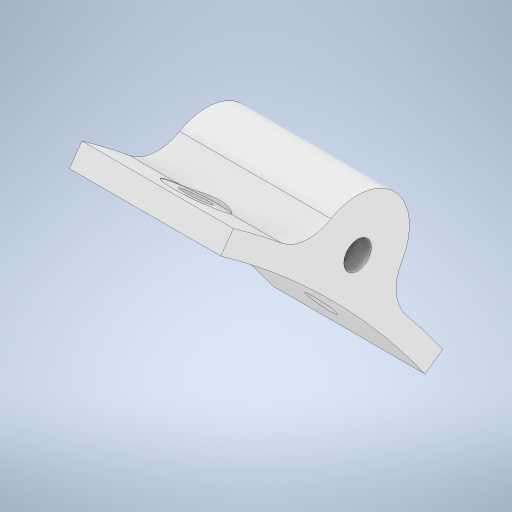
# Autodesk Inventor part: Lüfterhalter
Saved by Autodesk Inventor 2023 (Build 270158000, 158)
## iProperties
Created: 2023-01-25
Part Number: Lüfterhalter
Material: Generisch
Document SubType Name: Modeling
Designer: prigge
Density: 1 g/cm^3
Appearance: Glatt - Weiß
Author: prigge
Autodesk Inventor part; units mm, degrees
ref_plane "XY Plane" through (0, 0, 0) normal (0, 0, 1) x (1, 0, 0)
sketch "Skizze1" plane through (0, 0, 0) normal (1, 0, 0) x (0, 1, 0)
  line L0 (0, 0) -> (147.4318, -147.4318) construction
  line L1 (0, 33.4705) -> (0, -200.8229) construction
  circle A0 centre (147.4318, -147.4318) radius 3.2
  line L2 (0, 0) -> (156.5216, -124.5029) construction
  line L3 (-33.4705, 0) -> (200.8229, 0) projected
  arc A1 (115.8562, -163.0256) -> (163.0256, -115.8562) centre (0, 0) ccw
  line L4 (0, 0) -> (163.0256, -115.8562) construction
  line L5 (163.0256, -115.8562) -> (167.1012, -118.7526)
  arc A2 (152.7783, -136.6887) -> (167.1012, -118.7526) centre (0, 0) ccw
  arc A3 (118.7526, -167.1012) -> (136.6887, -152.7783) centre (0, 0) ccw
  arc A4 (136.6887, -152.7783) -> (152.7783, -136.6887) centre (147.4318, -147.4318) ccw
  line L6 (115.8562, -163.0256) -> (118.7526, -167.1012)
  dimension "d0" = 45
  dimension "d1" = 208.5
  dimension "d2" = 6.4
  dimension "d3" = 38.5
  dimension "d4" = 200
  dimension "d5" = 54.6
  dimension "d6" = 5
  dimension "d7" = 12
  constraints: 10 end point, 10 point on circle, 5 centre point, 3 coincident, 3 symmetric about line, 2 point on line, 1 collinear, 1 other
  measures "d0" angle of L1 L0
  measures "d1" distance of L0.start L0.end
  measures "d2" diameter of A0
  measures "d3" angle of L3 L2
  measures "d4" radius of A1
  measures "d5" angle of L1 L4
  measures "d6" distance of L4.end L5.end
  measures "d7" radius of A4
extrude "Extrusion1" add sketch "Skizze1" against normal blind 35
fillet "Rundung1" radius 10 2 edges at (-17.5, 136.6887, -152.7783) (-17.5, 152.7783, -136.6887)
ref_plane "Arbeitsebene1" through (-17.5, 0, 0) normal (1, 0, 0) x (0, 1, 0)
sketch "Skizze2" plane through (-17.5, 0, 0) normal (1, 0, 0) x (0, 1, 0)
  line L0 (0, 0) -> (141.692, -178.1312) construction
  line L1 (0, -213.7575) -> (0, 35.6262) projected
  line L2 (124.487, -156.5016) -> (121.9826, -158.4936)
  arc A0 (115.8562, -163.0256) -> (163.0256, -115.8562) centre (0, 0) ccw projected
  line L3 (121.9826, -158.4936) -> (125.047, -162.3461)
  arc A1 (118.7526, -167.1012) -> (129.8706, -158.6147) centre (0, 0) ccw projected
  line L4 (125.047, -162.3461) -> (122.4644, -164.4004)
  line L5 (122.4644, -164.4004) -> (125.577, -168.3134)
  line L6 (125.577, -168.3134) -> (130.6639, -164.267)
  line L7 (124.487, -156.5016) -> (130.6639, -164.267)
  point P0 (124.5029, -156.5216)
  dimension "d12" = 38.5
  dimension "d13" = 5
  dimension "d14" = 6.4
  dimension "d15" = 13
  constraints: 14 end point, 4 perpendicular, 2 point on circle, 2 point on line, 1 collinear, 1 parallel
  measures "d12" angle of L1 L0
  measures "d13" distance of L4.end L5.end
  measures "d14" diameter of L3 L0
  measures "d15" diameter of L5 L0
revolve "Umdrehung1" cut sketch "Skizze2" angle 360 about axis through (-17.5, 0, 0) along (0, 0.6225146, -0.7826082) contours A0 L7 A1 L4 L3 | L7 L6 L5 A1
ref_plane "Arbeitsebene2" through (0, 0, 0) normal (0, 0.7071068, 0.7071068) x (1, 0, 0)
mirror "Spiegeln1" about plane through (0, 0, 0) normal (0, 0.7071068, 0.7071068) of "Umdrehung1"
sketch "Skizze4" plane through (0, 0, 0) normal (1, 0, 0) x (0, 0, -1)
  line L0 (115.8562, 163.0256) -> (118.7526, 167.1012) projected
  circle A0 centre (118.7526, 167.1012) radius 2
  circle A1 centre (115.8562, 163.0256) radius 2
  line L1 (167.1012, 118.7526) -> (163.0256, 115.8562) projected
  circle A2 centre (167.1012, 118.7526) radius 2
  circle A3 centre (163.0256, 115.8562) radius 2
  point P0 (0, 0)
  dimension "d18" = 4
  constraints: 4 centre point, 3 equal radius, 2 coincident
  measures "d18" diameter of A0
